Moyeu 6 Hex 12 (Autodesk Fusion 360 design; units mm, degrees)
Autodesk Fusion 360 part; units mm, degrees
note: some values were not read from the file. Chosen so that the rebuilt part matches the saved one: a direction; which face or edge a step refers to. Set by a fixed rule: which sketch regions a step uses.
sketch "Sketch1" plane through (0, 0, 0) normal (0, 0, 1) x (1, 0, 0)
  line L0 (6.261, -2.9665) -> (5.6995, 3.9389)
  line L1 (5.6995, 3.9389) -> (-0.5615, 6.9054)
  line L2 (-0.5615, 6.9054) -> (-6.261, 2.9665)
  line L3 (-6.261, 2.9665) -> (-5.6995, -3.9389)
  line L4 (-5.6995, -3.9389) -> (0.5615, -6.9054)
  line L5 (0.5615, -6.9054) -> (6.261, -2.9665)
  dimension "d1" = 6
  measures "d1" distance of origin L5
extrude "Extrude1" add sketch "Sketch1" along normal blind 6
fillet "Fillet1" radius 0.2 8 faces at (-6.0738, 0.6647, 2) (3.6125, 4.9278, 2) (5.8867, 1.6371, 4) (2.087, -0.9888, 0) (-2.4613, 5.5924, 2) (2.4613, -5.5924, 2) (2.087, -0.9888, 6) (-3.6125, -4.9278, 2)
sketch "Sketch3" plane through (0, 0, 6) normal (0, 0, 1) x (-1, 0, 0)
  line L0 (6.0523, -2.8676) -> (5.5096, 3.8076)
  line L1 (5.5096, 3.8076) -> (-0.5427, 6.6752)
  line L2 (-0.5427, 6.6752) -> (-6.0523, 2.8676)
  line L3 (-6.0523, 2.8676) -> (-5.5096, -3.8076)
  line L4 (-5.5096, -3.8076) -> (0.5427, -6.6752)
  line L5 (0.5427, -6.6752) -> (6.0523, -2.8676)
  circle A0 centre (0, 0) radius 5.75
  circle A1 centre (0, 0) radius 3
  circle A2 centre (0, 0) radius 1.5
  dimension "d10" = 11.5
  dimension "d11" = 6
  dimension "d14" = 3
  constraint coincident A0.centre A1.centre
  constraint concentric A0 A1
  constraint concentric A1 A2
  measures "d10" diameter of A0
  measures "d11" diameter of A1
  measures "d14" diameter of A2
extrude "Extrude3" add sketch "Sketch3" along normal blind 12 contours A0
extrude "Extrude4" cut sketch "Sketch3" against normal through all contours A2
fillet "Fillet2" radius 0.2 2 edges at (2.797, -1.0848, 18) (5.3609, 2.0793, 18)
